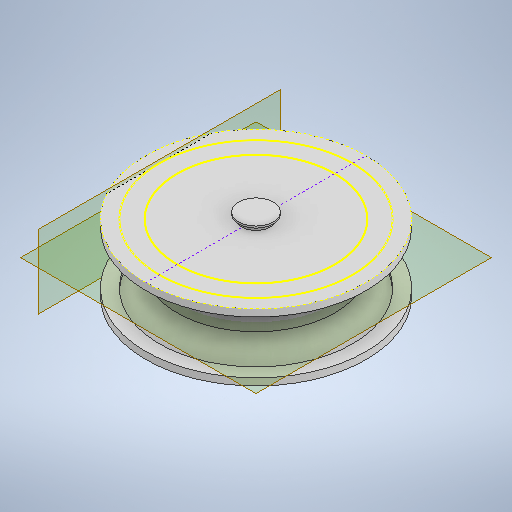
# Autodesk Inventor part: WireRewindDRUM
Saved by Autodesk Inventor 2025.1 (Build 291241000, 241)
## iProperties
Created: 2024-10-25
Part Number: WireRewindDRUM
Material: Generic
Document SubType Name: Modeling
Designer: ishaa
Density: 1 g/cm^3
Appearance: Default
Author: ishaa
Autodesk Inventor part; units mm, degrees
ref_plane "YZ Plane" through (0, 0, 0) normal (1, 0, 0) x (0, 1, 0)
ref_plane "XZ Plane" through (0, 0, 0) normal (0, 1, 0) x (-1, 0, 0)
ref_plane "XY Plane" through (0, 0, 0) normal (0, 0, 1) x (1, 0, 0)
sketch "Sketch1" plane through (0, 0, 0) normal (0, 0, 1) x (1, 0, 0)
  line L0 (0, 0) -> (27.5, 0)
  line L1 (27.5, 17) -> (0, 17)
  line L2 (0, 17) -> (0, 0)
  line L3 (0, 8.5) -> (32.996, 8.5) construction
  line L4 (27.5, 17) -> (20.3677, 8.5)
  line L5 (27.5, 17) -> (38.596, 17) construction
  line L6 (27.5, 0) -> (20.3677, 8.5)
  dimension "d0" = 27.5
  dimension "d2" = 17
  dimension "d3" = 27.5
  dimension "d4" = 130
  constraints: 14 end point, 3 horizontal, 1 equal length, 1 midpoint, 1 parallel, 1 perpendicular, 1 point on line
  measures "d0" distance of L1.end L1.start
  measures "d2" distance from line of L0.start L1
  measures "d3" distance from line of L0.end L2
  measures "d4" angle of L4 L5
revolve "Revolution1" add sketch "Sketch1" angle 360 about axis through (0, 17, 0) along (0, -1, 0)
sketch "Sketch4" plane through (0, 0, 0) normal (0, -1, 0) x (1, 0, 0)
  circle A0 centre (0, 0) radius 27.5 projected
  circle A1 centre (0, 0) radius 31.31
  dimension "d12" = 3.81
  constraints: 1 centre point
  measures "d12" radial gap between concentric circles of A0 A1
extrude "Extrusion2" add sketch "Sketch4" along normal blind 1 and the other way blind 1
ref_plane "Work Plane1" through (0, 8.5, 0) normal (0, -1, 0) x (1, 0, 0)
sketch "Sketch5" plane through (0, 0, 0) normal (0, -1, 0) x (1, 0, 0)
  circle A0 centre (0, 0) radius 27.5
  constraints: 1 centre point, 1 coincident
extrude "Extrusion3" add sketch "Sketch5" along normal blind 1
mirror "Mirror1" about plane through (0, 8.5, 0) normal (0, -1, 0) of "Extrusion2"
sketch "Sketch6" plane through (0, 17, 0) normal (0, 1, 0) x (1, 0, 0)
  circle A0 centre (0, 0) radius 27.5
  constraints: 1 centre point, 1 coincident
extrude "Extrusion4" add sketch "Sketch6" along normal blind 1
chamfer "Chamfer1" distance 3.175 angle 45 1 edges at (-20.3677, 8.5, 0)
sketch "Sketch7" plane through (0, 18, 0) normal (0, 1, 0) x (1, 0, 0)
  circle A0 centre (0, 0) radius 31.31 construction
  line L0 (0, 31.31) -> (0, -31.31) construction
  circle A1 centre (0, 0) radius 22.4085 projected
  circle A2 centre (0, 0) radius 27.5 projected
  circle A3 centre (0, 0) radius 22.4085 projected
  circle A4 centre (0, 0) radius 27.5 construction
  line L1 (-27.5, 14.9688) -> (-27.5, 0) construction
  circle A5 centre (0, 0) radius 27.5 construction
  line L2 (-27.5, -14.9688) -> (-27.5, 0) construction
  constraints: 6 end point, 4 point on circle, 4 vertical, 2 tangent, 1 horizontal alignment, 1 other
ref_plane "Work Plane2" through (-27.5, 18, 14.9688) normal (-1, 0, 0) x (0, 0, -1)
sketch "Sketch8" plane through (-27.5, 18, 14.9688) normal (-1, 0, 0) x (0, 0, -1)
  line L0 (37.3773, 7.0678) -> (37.3773, 11.9322) construction
  line L1 (37.3773, 9.5) -> (-7.4397, 9.5) construction
  line L2 (-7.4397, 7.0678) -> (-7.4397, 11.9322) construction
  line L3 (18.361, 15.7245) -> (11.5766, 15.7245)
  line L4 (11.5766, 15.7245) -> (11.5766, 3.2755)
  line L5 (11.5766, 3.2755) -> (18.361, 3.2755)
  line L6 (18.361, 3.2755) -> (18.361, 15.7245)
  line L7 (18.361, 15.7245) -> (11.5766, 3.2755) construction
  line L8 (11.5766, 15.7245) -> (18.361, 3.2755) construction
  point P0 (14.9688, 18)
  point P1 (14.9688, 9.5)
  constraints: 14 end point, 5 midpoint, 2 parallel, 1 horizontal, 1 perpendicular
extrude "Extrusion5" add sketch "Sketch8" along normal blind 3 and the other way blind 5
chamfer "Chamfer2" distance 3.175 angle 45 1 edges at (-30.5, 8.5, 3.3922)
sketch "Sketch9" plane through (-25.3648, 2.2755, -3.3922) normal (0, 0, -1) x (-1, 0, 0)
  line L0 (5.1352, 0) -> (1.9602, 0) projected
  line L1 (0, 12.449) -> (5.1352, 12.449) projected
  line L2 (3.5477, 0) -> (5.1352, 0)
  line L3 (5.1352, 0) -> (5.1352, 12.449)
  line L4 (5.1352, 12.449) -> (3.5477, 12.449)
  line L5 (3.5477, 12.449) -> (3.5477, 0)
  point P0 (-25.3648, -2.2755)
  constraints: 8 end point, 2 parallel, 1 horizontal, 1 midpoint, 1 perpendicular
extrude "Extrusion6" add sketch "Sketch9" along normal blind 4.5
fillet "Fillet2" radius 3.175 1 edges at (-28.9125, 8.5, -3.3922)
sketch "Sketch10" plane through (0, 18, 0) normal (0, 1, 0) x (1, 0, 0)
  circle A0 centre (0, 0) radius 4
  dimension "d35" = 8
  constraints: 1 centre point, 1 coincident
  measures "d35" diameter of A0
extrude "Extrusion7" add sketch "Sketch10" along normal blind 1.5
sketch "Sketch11" plane through (0, 19.5, 0) normal (0, 1, 0) x (1, 0, 0)
  circle A0 centre (0, 0) radius 4.9245
  dimension "d38" = 9.849
  constraints: 1 centre point, 1 coincident
  measures "d38" diameter of A0
extrude "Extrusion8" add sketch "Sketch11" along normal mid plane 0.5
body "Solid1"
